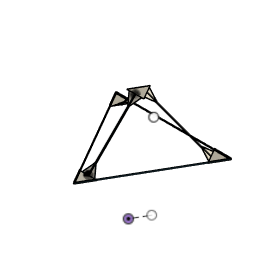
R-OSE Platform (Autodesk Fusion 360 design; units mm, degrees)
Autodesk Fusion 360 part; units mm, degrees
sketch "Esquisse1" plane through (0, 0, 0) normal (0, 0, 1) x (1, 0, 0)
  line L0 (0, 0) -> (-150, 0)
  line L1 (-150, 0) -> (-75, 129.9038)
  line L2 (-75, 129.9038) -> (0, 0)
  dimension "d1" = 150
  dimension "d2" = 60
  dimension "d3" = 150
  constraint horizontal L0
  constraint coincident L0.start L2.end
  measures "d1" distance of L0.start L0.end
  measures "d2" angle of L0 L1
  measures "d3" distance of L0.end L1.end
extrude "Extrusion1" add sketch "Esquisse1" along normal blind 1 makes body 1
sketch "Esquisse2" plane through (0, 0, 1) normal (0, 0, 1) x (-1, 0, 0)
  line L0 (75, -129.9038) -> (150, 0)
  line L1 (150, 0) -> (0, 0)
  line L2 (0, 0) -> (75, -129.9038)
  line L3 (6.928, 0) -> (1006.928, 0)
  line L4 (1006.928, 0) -> (1006.928, -4)
  line L5 (1006.928, -4) -> (6.928, -4)
  line L6 (6.928, -4) -> (6.928, 0)
  dimension "d6" = 1000
  dimension "d7" = 6.928
  dimension "d8" = 4
  dimension "d9" = 1000
  constraint coincident L1 L3.start
  constraint vertical L4
  constraint perpendicular L4 L5
  constraint perpendicular L3 L6
  measures "d6" distance of L3.start L3.end
  measures "d7" distance of L1.end L3.start
  measures "d8" distance of L3.end L4.end
  measures "d9" distance of L4.end L5.end
extrude "Extrusion2" add sketch "Esquisse2" along normal blind 4 separate body contours L0 L1 L3 L5 L6 | L0 L3 L4 L5 makes body 2
sketch "Esquisse3" plane through (-6.928, 0, 0) normal (1, 0, 0) x (0, 1, 0)
  line L0 (4, 1) -> (4, 5)
  line L1 (4, 5) -> (0, 5)
  line L2 (0, 5) -> (0, 1)
  circle A0 centre (2, 3) radius 1.25
  line L3 (0, 1) -> (4, 1)
  dimension "d12" = 2
  dimension "d13" = 2
  dimension "d14" = 2.5
  measures "d12" distance of L1 A0.centre
  measures "d13" distance of L0 A0.centre
  measures "d14" diameter of A0
extrude "Extrusion3" cut sketch "Esquisse3" against normal blind 1000 contours A0 bodies 2
sketch "Esquisse4" plane through (0, 0, 0) normal (0, -1, 0) x (1, 0, 0)
  line L0 (-150, 0) -> (0, 0)
  line L1 (0, 0) -> (0, 1)
  line L2 (0, 1) -> (-150, 1)
  line L3 (-6.928, 1) -> (-6.928, 5)
  line L4 (-6.928, 5) -> (-1006.928, 5)
  line L5 (-1006.928, 5) -> (-1006.928, 1)
  line L6 (-1006.928, 1) -> (-6.928, 1)
  line L7 (-150, 1) -> (-150, 0)
  line L8 (0, 0) -> (-150, 0)
  line L9 (-150, 0) -> (-150, 10)
  line L10 (-150, 10) -> (0, 10)
  line L11 (0, 10) -> (0, 0)
  dimension "d17" = 10
  constraint coincident L0.end L1.start
  constraint coincident L0.start L7.end
  constraint perpendicular L4 L9
  constraint perpendicular L9 L10
  constraint perpendicular L8 L11
  measures "d17" distance of L0.start L9.end
extrude "Extrusion4" add sketch "Esquisse4" along normal blind 1 separate body contours L0 L1 L2 L6 L7 L8 L9 L11 | L2 L3 L4 L6 L9 | L2 L3 L4 L9 L10 L11 makes body 3
sketch "Esquisse5" plane through (0, 0, 0) normal (0.866025, 0.5, 0) x (-0.5, 0.866025, 0)
  line L0 (0, 0) -> (150, 0)
  line L1 (150, 0) -> (150, 1)
  line L2 (150, 1) -> (0, 1)
  line L3 (0, 0) -> (0, 10)
  line L4 (0, 10) -> (125, 10)
  line L5 (125, 10) -> (150, 10)
  line L6 (150, 10) -> (150, 0)
  line L7 (0, 1) -> (0, 0)
  constraint coincident L0.start L3.start
  constraint perpendicular L2 L3
  constraint perpendicular L3 L4
  constraint perpendicular L1 L5
  constraint coincident L0.end L1.start
  constraint perpendicular L5 L6
extrude "Extrusion5" add sketch "Esquisse5" along normal blind 1 bodies 2 1 3
ref_plane "Plan de construction1" through (-112.5, 64.9519, 0) normal (0.612372, -0.353553, 0.707107) x (0.5, 0.866025, 0)
sketch "Esquisse6" plane through (-112.5, 64.9519, 0) normal (0.612372, -0.353553, 0.707107) x (0.5, 0.866025, 0)
  line L0 (0, 0) -> (55, 0)
  line L1 (0, 0) -> (-55, 0)
  line L2 (-55, 0) -> (0, 95.2628)
  line L3 (55, 0) -> (0, 95.2628)
  dimension "d23" = 55
  dimension "d24" = 55
  dimension "d25" = 60
  dimension "d26" = 110
  constraint coincident L0.start L1.start
  constraint horizontal L0
  constraint horizontal L1
  measures "d23" distance of L0.start L0.end
  measures "d24" distance of L0.start L1.end
  measures "d25" angle of L1 L2
  measures "d26" distance of L1.end L2.end
extrude "Extrusion6" add sketch "Esquisse6" along normal blind 1 bodies 2 1
pattern_linear "Réseau R1" count 1 spacing 0 along (1, 0, 0) count 3 spacing 450 along (0, 1, 0) of bodies 2 1 makes body 4 at (-75, 493.3013, 0) makes body 5 at (-75, 943.3013, 0) makes body 6 at (-673.5947, 453.0825, 3.625) makes body 7 at (-673.5947, 903.0825, 3.625)
move_body "Aligner1" bodies 4 to x (0.5, -0.866025, 0) y (0.866025, 0.5, 0) z (0, 0, 1) at (-588.0313, 110.5001, 0)
copy_body "Corps->Comp1" bodies 1 removing the originals makes body 8 in component "Triangle 1"
copy_body "Corps->Comp2" bodies 5 removing the originals makes body 9 in component "Triangle 2"
copy_body "Corps->Comp3" bodies 4 removing the originals makes body 10 in component "Triangle 3"
copy_body "Corps->Comp5" bodies 2 removing the originals makes body 11 in component "Tige 1"
copy_body "Corps->Comp6" bodies 6 removing the originals makes body 12 in component "Tige 2"
copy_body "Corps->Comp7" bodies 7 removing the originals makes body 13 in component "Tige 3"
sketch "Esquisse28" plane through (-709.7424, -411.425, -72.2462) normal (0.612372, 0.353553, -0.707107) x (-0.5, 0.866025, 0)
  line L0 (453.3613, 102.1716) -> (563.3613, 102.1716)
  line L1 (563.3613, 102.1716) -> (508.3613, 197.4343)
  line L2 (508.3613, 197.4343) -> (453.3613, 102.1716)
  line L3 (508.3613, 102.1716) -> (506.3613, 102.1716)
  line L4 (506.3613, 102.1716) -> (506.3613, 691.9135)
  line L5 (506.3613, 691.9135) -> (510.3613, 691.9135)
  line L6 (510.3613, 691.9135) -> (510.3613, 102.1716)
  line L7 (510.3613, 102.1716) -> (506.3613, 102.1716)
  dimension "d223" = 2
  dimension "d224" = 589.7419
  dimension "d225" = 4
  constraint midpoint L0 L3.start
  constraint parallel L0 L3
  constraint perpendicular L0 L4
  constraint perpendicular L4 L5
  constraint coincident L0 L6.end
  constraint perpendicular L0 L6
  measures "d223" distance of L3.start L3.end
  measures "d224" distance of L3.end L4.end
  measures "d225" distance of L4.end L5.end
sketch "Esquisse29" plane through (-770.4847, 577.8446, -595.2298) normal (-0.612372, 0.353553, 0.707107) x (0.5, 0.866025, 0)
  line L0 (219.609, -850.2673) -> (329.609, -850.2673)
  line L1 (329.609, -850.2673) -> (274.609, -755.0045)
  line L2 (274.609, -755.0045) -> (219.609, -850.2673)
  line L3 (274.609, -850.2673) -> (276.609, -850.2673)
  line L4 (276.609, -850.2673) -> (276.609, -260.5253)
  line L5 (276.609, -260.5253) -> (272.609, -260.5253)
  line L6 (272.609, -260.5253) -> (272.609, -850.2673)
  line L7 (276.609, -850.2673) -> (272.609, -850.2673)
  dimension "d228" = 2
  dimension "d229" = 589.7419
  dimension "d230" = 4
  constraint midpoint L0 L3.start
  constraint coincident L0 L3.end
  constraint perpendicular L3 L4
  constraint perpendicular L4 L5
  constraint coincident L0 L6.end
  constraint perpendicular L0 L6
  measures "d228" distance of L3.start L3.end
  measures "d229" distance of L3.end L4.end
  measures "d230" distance of L4.end L5.end
sketch "Esquisse31" plane through (0, 77.9393, -77.9393) normal (0, -0.707107, 0.707107) x (-1, 0, 0)
  line L0 (451.9279, -110.2228) -> (561.9279, -110.2228)
  line L1 (561.9279, -110.2228) -> (506.9279, -205.4856)
  line L2 (506.9279, -205.4856) -> (451.9279, -110.2228)
  line L3 (506.9279, -110.2228) -> (506.9279, -690.2228) construction
  line L4 (506.9279, -690.2228) -> (504.9279, -690.2228)
  line L5 (504.9279, -690.2228) -> (504.9279, -110.2228)
  line L6 (504.9279, -110.2228) -> (506.9279, -110.2228)
  line L7 (508.9279, -110.2228) -> (506.9279, -110.2228)
  line L8 (508.9279, -690.2228) -> (508.9279, -110.2228)
  line L9 (506.9279, -690.2228) -> (508.9279, -690.2228)
  dimension "d258" = 580
  dimension "d259" = 2
  dimension "d260" = 90
  constraint midpoint L0 L3.start
  constraint perpendicular L0 L3
  constraint perpendicular L3 L4
  constraint coincident L0 L5.end
  constraint symmetric L6.end L3 L7.end
  constraint symmetric L4.start L3 L9.start
  constraint symmetric L3 L4.end L8.start
  constraint symmetric L3 L5.end L7.start
  measures "d258" distance of L3.start L3.end
  measures "d259" distance of L3.end L4.end
  measures "d260" angle of L4 L5
extrude "Extrusion22" add sketch "Esquisse31" against normal blind 4 separate body contours L0 L1 L2 L5 L6 L7 L8 | L1 L2 L4 L5 L8 L9 makes body 14
copy_body "Corps->Comp12" bodies 14 removing the originals makes body 15 in component "Tige 4"
sketch "Esquisse32" plane through (0, 77.9393, 77.9393) normal (0, -0.707107, -0.707107) x (1, 0, 0)
  line L0 (-504.9279, -110.2228) -> (-508.9279, -110.2228)
  line L1 (-508.9279, -110.2228) -> (-508.9279, -114.2228)
  line L2 (-508.9279, -114.2228) -> (-504.9279, -114.2228)
  line L3 (-504.9279, -114.2228) -> (-504.9279, -110.2228)
  circle A0 centre (-506.9279, -112.2228) radius 1.25
  dimension "d265" = 2.5
  dimension "d266" = 2
  dimension "d267" = 2
  measures "d265" diameter of A0
  measures "d266" distance of L2 A0.centre
  measures "d267" distance of L3 A0.centre
extrude "Extrusion1'" cut sketch "Esquisse32" against normal through all contours A0 bodies 15 in component "Tige 4"
sketch "Esquisse33" plane through (139.4717, 80.524, 161.0481) normal (-0.612372, -0.353553, -0.707107) x (0.5, -0.866025, 0)
  line L0 (-837.8868, -227.7564) -> (-727.8868, -227.7564)
  line L1 (-727.8868, -227.7564) -> (-782.8868, -132.4936)
  line L2 (-782.8868, -132.4936) -> (-837.8868, -227.7564)
  line L3 (-780.8868, -227.7564) -> (-784.8868, -227.7564)
  line L4 (-780.8868, -227.7564) -> (-784.8868, -227.7564)
  line L5 (-784.8868, -227.7564) -> (-784.8868, 352.2436)
  line L6 (-784.8868, 352.2436) -> (-780.8868, 352.2436)
  line L7 (-780.8868, 352.2436) -> (-780.8868, -227.7564)
  point P0 (-782.8868, -227.7564)
  dimension "d269" = 4
  dimension "d270" = 4
  dimension "d271" = 580
  constraint midpoint L0 P0
  constraint coincident L0 L3.start
  constraint parallel L0 L3
  constraint midpoint P0 L3
  constraint horizontal L4
  constraint vertical L5
  constraint horizontal L6
  constraint vertical L7
  measures "d269" distance of L3.start L3.end
  measures "d270" distance of L3.start L3.end
  measures "d271" distance of L3.start L6.end
extrude "Extrusion1''" add sketch "Esquisse33" along normal blind 4 separate body contours L0 L1 L2 L3 L4 L5 L7 | L1 L2 L5 L6 L7 makes body 16 in component "Tige 5"
sketch "Esquisse34" plane through (139.4717, 80.524, -161.0481) normal (0.612372, 0.353553, -0.707107) x (-0.5, 0.866025, 0)
  line L0 (784.8868, 227.7564) -> (780.8868, 227.7564)
  line L1 (780.8868, 227.7564) -> (780.8868, 223.7564)
  line L2 (780.8868, 223.7564) -> (784.8868, 223.7564)
  line L3 (784.8868, 223.7564) -> (784.8868, 227.7564)
  circle A0 centre (782.8868, 225.7564) radius 1.25
  dimension "d274" = 2.5
  dimension "d275" = 2
  dimension "d276" = 2
  measures "d274" diameter of A0
  measures "d275" distance of L2 A0.centre
  measures "d276" distance of L1 A0.centre
extrude "Extrusion2'" cut sketch "Esquisse34" along normal through all and the other way through all contours A0 bodies 16 in component "Tige 5"
sketch "Esquisse36" plane through (-519.6677, 300.0303, 600.0606) normal (0.612372, -0.353553, -0.707107) x (0.5, 0.866025, 0)
  line L0 (220.959, -848.6139) -> (330.959, -848.6139)
  line L1 (330.959, -848.6139) -> (275.959, -753.3511)
  line L2 (275.959, -753.3511) -> (220.959, -848.6139)
  line L3 (273.959, -848.6139) -> (277.959, -848.6139)
  line L4 (273.959, -848.6139) -> (277.959, -848.6139)
  line L5 (277.959, -848.6139) -> (277.959, -268.6139)
  line L6 (277.959, -268.6139) -> (273.959, -268.6139)
  line L7 (273.959, -268.6139) -> (273.959, -848.6139)
  point P0 (275.959, -848.6139)
  dimension "d297" = 4
  dimension "d298" = 4
  dimension "d299" = 580
  constraint midpoint L0 P0
  constraint coincident L0 L3.start
  constraint parallel L0 L3
  constraint midpoint P0 L3
  constraint horizontal L4
  constraint vertical L5
  constraint horizontal L6
  constraint vertical L7
  measures "d297" distance of L3.start L3.end
  measures "d298" distance of L3.start L3.end
  measures "d299" distance of L3.start L6.end
extrude "Extrusion1'''" add sketch "Esquisse36" along normal blind 4 separate body contours L0 L1 L2 L3 L4 L5 L7 | L1 L2 L5 L6 L7 makes body 17 in component "Tige 6"
sketch "Esquisse37" plane through (-519.6677, 300.0303, -600.0606) normal (-0.612372, 0.353553, -0.707107) x (-0.5, -0.866025, 0)
  line L0 (-273.959, 848.6139) -> (-277.959, 848.6139)
  line L1 (-277.959, 848.6139) -> (-277.959, 844.6139)
  line L2 (-277.959, 844.6139) -> (-273.959, 844.6139)
  line L3 (-273.959, 844.6139) -> (-273.959, 848.6139)
  circle A0 centre (-275.959, 846.6139) radius 1.25
  dimension "d306" = 2
  dimension "d307" = 2
  dimension "d308" = 2.5
  measures "d306" distance of L2 A0.centre
  measures "d307" distance of L3 A0.centre
  measures "d308" diameter of A0
extrude "Extrusion2''" cut sketch "Esquisse37" along normal through all and the other way through all contours A0 bodies 17 in component "Tige 6"
sketch "Esquisse38" plane through (0, 0, 0) normal (0, 0, 1) x (1, 0, 0)
  line L0 (0, 0) -> (150, 0)
  line L1 (150, 0) -> (75, 129.9038)
  line L2 (75, 129.9038) -> (0, 0)
  dimension "d311" = 150
  dimension "d312" = 60
  constraint coincident L0.start L2.end
  constraint horizontal L0
  measures "d311" distance of L0.end L1.end
  measures "d312" angle of L0 L1
extrude "Extrusion24" add sketch "Esquisse38" along normal blind 1 separate body makes body 18
copy_body "Corps->Comp14" bodies 18 removing the originals makes body 19 in component "Base"
ref_plane "Plan de construction5" through (75, 0, 1) normal (0, -0.707107, 0.707107) x (1, 0, 0)
sketch "Esquisse40" plane through (0, -0.5, 0.5) normal (0, -0.707107, 0.707107) x (1, 0, 0)
  line L0 (130, 0.7071) -> (20, 0.7071)
  line L1 (0, 0.7071) -> (150, 0.7071)
  line L2 (130, 0.7071) -> (75, -94.5557)
  line L3 (130, 0.7071) -> (240, 0.7071) construction
  line L4 (75, -94.5557) -> (20, 0.7071)
  point P0 (149.7264, -579.2928)
  point P1 (150, 0.7071)
  dimension "d317" = 110
  dimension "d318" = 20
  dimension "d319" = 120
  dimension "d320" = 110
  constraint horizontal L0
  constraint collinear L0 L1
  constraint horizontal L3
  measures "d317" distance of L0.start L0.end
  measures "d318" distance of L0.end L1.start
  measures "d319" angle of L2 L3
  measures "d320" distance of L0.start L2.end
extrude "Extrusion1''''" add sketch "Esquisse40" against normal blind 1 bodies 19 in component "Base"
ref_plane "Plan de construction7" through (37.5, 64.9519, 1) normal (-0.612372, 0.353553, 0.707107) x (-0.5, -0.866025, 0)
sketch "Esquisse44" plane through (-0.433, 0.25, 0.5) normal (-0.612372, 0.353553, 0.707107) x (-0.5, -0.866025, 0)
  line L0 (0, 0) -> (-150, 0) construction
  constraint coincident L0.start origin
  constraint horizontal L0
sketch "Esquisse45" plane through (-0.433, 0.25, 0.5) normal (-0.612372, 0.353553, 0.707107) x (-0.5, -0.866025, 0)
  line L0 (0, 0.707) -> (-150, 0.707) construction
  line L1 (-150, 0.707) -> (-130, 0.707)
  line L2 (-130, 0.707) -> (-75, -94.5558)
  line L3 (-130, 0.707) -> (-20, 0.707) construction
  line L4 (-75, -94.5558) -> (-20, 0.707)
  line L5 (-75, -94.5558) -> (35, -94.5558) construction
  line L6 (-20, 0.707) -> (-130, 0.707)
  dimension "d339" = 150
  dimension "d340" = 20
  dimension "d341" = 60
  dimension "d342" = 110
  dimension "d343" = 60
  dimension "d344" = 110
  constraint horizontal L0
  constraint parallel L0 L1
  constraint horizontal L3
  constraint horizontal L5
  measures "d339" distance of L0.start L0.end
  measures "d340" distance of L0.end L1.end
  measures "d341" angle of L2 L3
  measures "d342" distance of L1.end L2.end
  measures "d343" angle of L4 L5
  measures "d344" distance of L2.end L3.end
extrude "Extrusion27" [suppressed]
extrude "Extrusion4'" add sketch "Esquisse45" against normal blind 1 bodies 19 in component "Base"
ref_plane "Plan de construction8" through (112.5, 64.9519, 1) normal (0.612372, 0.353553, 0.707107) x (-0.5, 0.866025, 0)
sketch "Esquisse46" plane through (56.683, 32.726, 65.4519) normal (0.612372, 0.353553, 0.707107) x (-0.5, 0.866025, 0)
  line L0 (-75, -91.1488) -> (-55, -91.1488) construction
  line L1 (-55, -91.1488) -> (0, -186.4116)
  line L2 (-55, -91.1488) -> (55, -91.1488) construction
  line L3 (0, -186.4116) -> (55, -91.1488)
  line L4 (55, -91.1488) -> (-55, -91.1488)
  dimension "d348" = 20
  dimension "d349" = 60
  dimension "d350" = 110
  constraint horizontal L0
  constraint horizontal L2
  measures "d348" distance of L0.start L0.end
  measures "d349" angle of L1 L2
  measures "d350" distance of L0.end L1.end
extrude "Extrusion3'" add sketch "Esquisse46" against normal blind 1 bodies 19 in component "Base"
sketch "Esquisse47" plane through (-391.4433, 225.9999, 0) normal (0.866025, -0.5, 0) x (0.5, 0.866025, 0)
  line L0 (-224.0411, 1) -> (775.9589, 1)
  line L1 (775.9589, 1) -> (775.9589, 5)
  line L2 (775.9589, 5) -> (-224.0411, 5)
  line L3 (-224.0411, 5) -> (-224.0411, 1)
  line L4 (281.1824, 413.6929) -> (285.5447, 413.6929)
  dimension "d367" = 412.6929
  constraint horizontal L4
  measures "d367" distance of L0 L4
component "Triangle 1" placed x (0.5, 0.866025, 0) y (-0.866025, 0.5, 0) z (0, 0, 1) at (0.0001, 903.9998, 0)
component "Triangle 2" placed x (0.5, -0.866025, 0) y (0.866025, 0.5, 0) z (0, 0, 1) at (-1286.3508, -424.0252, 0)
component "Triangle 3" placed x (-0.5, -0.866025, 0) y (0.866025, -0.5, 0) z (0, 0, 1) at (-1403.5675, 900, 0)
component "Tige 1" placed x (0.5, 0.866025, 0) y (-0.866025, 0.5, 0) z (0, 0, 1) at (0.0001, 903.9998, 0)
component "Tige 2" placed x (-0.5, 0.866025, 0) y (0.866025, 0.5, 0) z (0, 0, -1) at (-1403.6507, 678.9519, 6)
component "Tige 3" placed x (1, 0, 0) y (0, 1, 0) z (0, 0, 1) at (0, 0, 0)
component "Tige 4" placed x (1, 0, 0) y (0, 1, 0) z (0, 0, 1) at (0, 0, 0)
component "Tige 5" placed x (1, 0, 0) y (0, 1, 0) z (0, 0, 1) at (0, 0, 0)
component "Tige 6" placed x (1, 0, 0) y (0, 1, 0) z (0, 0, 1) at (0, 0, 0)
component "Base" placed x (1, 0, 0) y (0, 1, 0) z (0, 0, 1) at (-581.9279, 568.0076, 412.5433)
equation "d204 = 150.00 mm - 6.928 mm"
equation "d217 = 75 mm - 6.928 mm"
equation "d224 = 500 mm - 0.5208652645 mm + 90.262794 mm"
equation "d229 = 500 mm - 0.5208652645 mm + 90.262794 mm"
equation "d243 = 150 mm - 6.928 mm"
